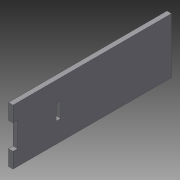
# Autodesk Inventor part: Back support
Saved by Autodesk Inventor 2015 (Build 190159000, 159)
## iProperties
Created: 2014-07-26
Part Number: Back support
Material: Generic
Document SubType Name: Modeling
Designer: karl
Density: 1 g/cm^3
Appearance: Default
Author: karl
Autodesk Inventor part; units mm, degrees
ref_plane "YZ Plane" through (0, 0, 0) normal (1, 0, 0) x (0, 1, 0)
ref_plane "XZ Plane" through (0, 0, 0) normal (0, 1, 0) x (-1, 0, 0)
ref_plane "XY Plane" through (0, 0, 0) normal (0, 0, 1) x (1, 0, 0)
sketch "Sketch1" plane through (0, 0, 0) normal (1, 0, 0) x (0, 1, 0)
  line L0 (-50, -18) -> (50, -18)
  line L1 (50, -18) -> (50, 18)
  line L2 (50, 18) -> (-50, 18)
  line L3 (-50, 18) -> (-50, -18)
  line L4 (-50, -18) -> (50, 18) construction
  line L5 (50, -18) -> (-50, 18) construction
  point P0 (0, 0)
  dimension "d0" = 36
  dimension "d1" = 100
  constraints: 12 end point, 2 midpoint, 2 parallel, 1 horizontal, 1 perpendicular
  measures "d0" distance of L1.end L0.end
  measures "d1" distance of L0.start L0.end
extrude "Extrusion1" add sketch "Sketch1" along normal blind 3
sketch "Sketch2" plane through (0, 0, 0) normal (-1, 0, 0) x (0, 0, 1)
  line L0 (-5, -22) -> (5, -22)
  line L1 (5, -22) -> (5, -25)
  line L2 (5, -25) -> (-5, -25)
  line L3 (-5, -25) -> (-5, -22)
  line L4 (18, -50) -> (-18, -50) projected
  point P0 (0, 0)
  point P1 (0, -22)
  dimension "d4" = 10
  dimension "d5" = 3
  dimension "d6" = 25
  constraints: 8 end point, 2 parallel, 1 horizontal, 1 midpoint, 1 perpendicular, 1 vertical alignment
  measures "d4" distance of L1.end L2.end
  measures "d5" distance of L0.end L1.end
  measures "d6" distance between parallel lines of L4 L2
extrude "Extrusion2" cut sketch "Sketch2" against normal blind 3
sketch "Sketch3" plane through (0, 0, 0) normal (-1, 0, 0) x (0, 0, 1)
  line L0 (-18, -50) -> (-8, -50)
  line L1 (-8, -50) -> (-8, -53)
  line L2 (-8, -53) -> (-18, -53)
  line L3 (-18, -53) -> (-18, -50)
  line L4 (18, -50) -> (8, -50)
  line L5 (8, -50) -> (8, -53)
  line L6 (8, -53) -> (18, -53)
  line L7 (18, -53) -> (18, -50)
  point P0 (0, 0)
  dimension "d9" = 10
  dimension "d10" = 3
  dimension "d11" = 10
  dimension "d12" = 3
  constraints: 16 end point, 4 parallel, 2 horizontal, 2 perpendicular
  measures "d9" distance of L1.end L2.end
  measures "d10" distance of L0.end L1.end
  measures "d11" distance of L6.end L5.end
  measures "d12" distance of L5.end L4.end
extrude "Extrusion3" add sketch "Sketch3" against normal blind 3
body "Solid1"
